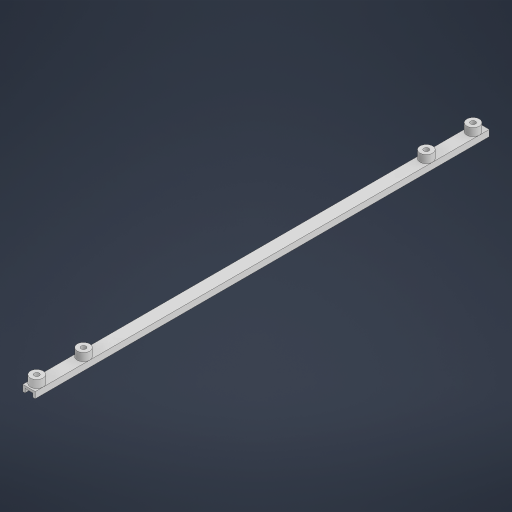
# Autodesk Inventor part: hs_intake_cb_jig
Saved by Autodesk Inventor 2024 (Build 280153000, 153)
## iProperties
Created: 2023-10-29
Part Number: hs_intake_cb_jig
Material: Generic
Document SubType Name: Modeling
Designer: Averey Ku
Density: 1 g/cm^3
Appearance: Default
Author: Averey Ku
Autodesk Inventor part; units mm, degrees
ref_plane "YZ Plane" through (0, 0, 0) normal (1, 0, 0) x (0, 1, 0)
ref_plane "XZ Plane" through (0, 0, 0) normal (0, 1, 0) x (-1, 0, 0)
ref_plane "XY Plane" through (0, 0, 0) normal (0, 0, 1) x (1, 0, 0)
sketch "Sketch1" plane through (0, 0, 0) normal (0, 0, 1) x (1, 0, 0)
  line L0 (3.175, 0) -> (3.175, 3.175)
  line L1 (3.175, 3.175) -> (-3.175, 3.175)
  line L2 (-3.175, 3.175) -> (-3.175, 0)
  line L3 (-5.08, 0) -> (-5.08, 5.08)
  line L4 (-5.08, 5.08) -> (5.08, 5.08)
  line L5 (5.08, 5.08) -> (5.08, 0)
  line L6 (5.08, 0) -> (3.175, 0)
  line L7 (-3.175, 0) -> (-5.08, 0)
  point P0 (0, 0)
  dimension "d0" = 10.16
  dimension "d1" = 5.08
  constraints: 16 end point, 4 parallel, 2 horizontal, 2 perpendicular
  measures "d0" distance of L3.end L4.end
  measures "d1" distance of L3.start L3.end
extrude "Extrusion1" add sketch "Sketch1" along normal blind 368.3
sketch "Sketch2" plane through (-5.08, 5.08, 0) normal (0, 1, 0) x (1, 0, 0)
  circle A0 centre (5.08, -6.35) radius 1.9844
  circle A1 centre (5.08, -44.45) radius 1.9844
  circle A2 centre (5.08, -361.95) radius 1.9844
  circle A3 centre (5.08, -323.85) radius 1.9844
  point P0 (5.08, 0)
  dimension "d4" = 3.9688
  dimension "d5" = 3.9688
  dimension "d6" = 3.9688
  dimension "d7" = 3.9688
  constraints: 4 centre point
  measures "d4" diameter of A0
  measures "d5" diameter of A1
  measures "d6" diameter of A2
  measures "d7" diameter of A3
extrude "Extrusion2" cut sketch "Sketch2" against normal blind 368.3
sketch "Sketch3" plane through (0, 0, 0) normal (0, 0, -1) x (-1, 0, 0)
  line L0 (-5.08, 0) -> (-5.08, 5.08) projected
  line L1 (5.08, 5.08) -> (-5.08, 5.08)
  line L2 (-5.08, 5.08) -> (-5.08, 0)
  line L3 (-5.08, 0) -> (5.08, 0)
  line L4 (5.08, 0) -> (5.08, 5.08)
  point P0 (0, 0)
  constraints: 8 end point, 2 parallel, 1 horizontal, 1 perpendicular
sketch "Sketch4" plane through (0, 0, 0) normal (0, 0, -1) x (-1, 0, 0)
  point P0 (0, 0)
extrude "Extrusion3" add sketch "Sketch3" along normal blind 1.778
sketch "Sketch5" plane through (-5.08, 5.08, 368.3) normal (0, 1, 0) x (1, 0, 0)
  circle A0 centre (5.08, 6.35) radius 1.9844 projected
  circle A1 centre (5.08, 44.45) radius 1.9844 projected
  circle A2 centre (5.08, 323.85) radius 1.9844 projected
  circle A3 centre (5.08, 361.95) radius 1.9844 projected
  circle A4 centre (5.08, 6.35) radius 5.08
  line L0 (10.16, 0) -> (10.16, 370.078) projected
  circle A5 centre (5.08, 44.45) radius 5.08
  circle A6 centre (5.08, 323.85) radius 5.08
  circle A7 centre (5.08, 361.95) radius 5.08
  point P0 (5.08, 368.3)
  constraints: 4 centre point, 4 coincident, 2 tangent
extrude "Extrusion4" add sketch "Sketch5" along normal blind 6.35
body "Solid1"
